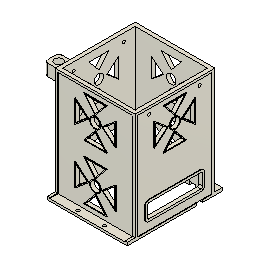
STRUCTURE-V1.0.1 (Autodesk Fusion 360 design; units mm, degrees)
Autodesk Fusion 360 part; units mm, degrees
note: some values were not read from the file. Set by a fixed rule: which sketch regions a step uses.
(part 1 of 2)
sketch "Sketch1" plane through (0, 0, 0) normal (0, 1, 0) x (1, 0, 0)
  line L0 (0, 0) -> (45, 0)
  line L1 (45, 0) -> (45, -45)
  line L2 (45, -45) -> (0, -45)
  line L3 (0, -45) -> (0, 0)
  line L4 (47.5, 2.5) -> (47.5, -47.5)
  line L5 (47.5, -47.5) -> (-2.5, -47.5)
  line L6 (-2.5, -47.5) -> (-2.5, 2.5)
  line L7 (-2.5, 2.5) -> (47.5, 2.5)
  dimension "d1" = 45
  dimension "d2" = 45
  dimension "d3" = -2.5
  constraint horizontal L0
  constraint vertical L1
  constraint horizontal L2
  constraint vertical L3
  constraint coincident L0.start L3.end
  measures "d1" distance of L0.start L0.end
  measures "d2" distance of L0.start L2.end
extrude "Extrude1" add sketch "Sketch1" along normal blind 70
sketch "Sketch2" plane through (0, 0, 47.5) normal (0, 0, 1) x (1, 0, 0)
  line L0 (-2.5, 0) -> (47.5, 0)
  line L1 (47.5, 0) -> (47.5, 70)
  line L2 (47.5, 70) -> (-2.5, 70)
  line L3 (-2.5, 70) -> (-2.5, 0)
  line L4 (-2.5, 35) -> (47.5, 35) construction
  circle A0 centre (22.5, 52.5) radius 3
  circle A1 centre (22.5, 17.5) radius 3
  line L5 (10, 65) -> (35, 65) construction
  line L6 (35, 65) -> (35, 40) construction
  line L7 (35, 40) -> (10, 40) construction
  line L8 (10, 40) -> (10, 65) construction
  line L9 (35, 52.5) -> (10, 52.5) construction
  line L10 (22.5, 65) -> (22.5, 40) construction
  line L11 (17.5, 57.5) -> (27.5, 57.5) construction
  line L12 (27.5, 57.5) -> (27.5, 47.5) construction
  line L13 (27.5, 47.5) -> (17.5, 47.5) construction
  line L14 (17.5, 47.5) -> (17.5, 57.5) construction
  line L15 (17.5, 22.5) -> (27.5, 22.5) construction
  line L16 (27.5, 22.5) -> (27.5, 12.5) construction
  line L17 (27.5, 12.5) -> (17.5, 12.5) construction
  line L18 (17.5, 12.5) -> (17.5, 22.5) construction
  line L19 (10, 30) -> (35, 30) construction
  line L20 (35, 30) -> (35, 5) construction
  line L21 (35, 5) -> (10, 5) construction
  line L22 (10, 5) -> (10, 30) construction
  line L23 (22.5, 57.5) -> (28.75, 65)
  line L24 (22.5, 57.5) -> (16.25, 65)
  line L25 (27.5, 52.5) -> (35, 58.75)
  line L26 (27.5, 52.5) -> (35, 46.25)
  line L27 (22.5, 47.5) -> (16.25, 40)
  line L28 (22.5, 47.5) -> (28.75, 40)
  line L29 (17.5, 52.5) -> (10, 58.75)
  line L30 (17.5, 52.5) -> (10, 46.25)
  line L31 (22.5, 22.5) -> (16.25, 30)
  line L32 (22.5, 22.5) -> (28.75, 30)
  line L33 (27.5, 17.5) -> (35, 23.75)
  line L34 (27.5, 17.5) -> (35, 11.25)
  line L35 (22.5, 12.5) -> (16.25, 5)
  line L36 (22.5, 12.5) -> (28.75, 5)
  line L37 (17.5, 17.5) -> (10, 23.75)
  line L38 (17.5, 17.5) -> (10, 11.25)
  line L39 (16.25, 65) -> (28.75, 65)
  line L40 (16.25, 5) -> (28.75, 5)
  line L41 (35, 11.25) -> (35, 23.75)
  line L42 (10, 23.75) -> (10, 11.25)
  line L43 (16.25, 30) -> (28.75, 30)
  line L44 (10, 46.25) -> (10, 58.75)
  line L45 (16.25, 40) -> (28.75, 40)
  line L46 (35, 46.25) -> (35, 58.75)
  line L47 (16.25, 65) -> (28.75, 65)
  dimension "d6" = 35
  dimension "d7" = 6
  dimension "d8" = 25
  dimension "d9" = 17.5
  dimension "d10" = 6
  dimension "d11" = 25
  dimension "d12" = 17.5
  dimension "d13" = 25
  dimension "d14" = 25
  dimension "d15" = 12.5
  dimension "d16" = 12.5
  dimension "d17" = 10
  dimension "d18" = 10
  dimension "d19" = 5
  dimension "d20" = 10
  dimension "d21" = 10
  dimension "d22" = 5
  dimension "d23" = 5
  dimension "d24" = 25
  dimension "d25" = 25
  dimension "d26" = 12.5
  dimension "d27" = 12.5
  dimension "d28" = 6.25
  dimension "d30" = 6.25
  dimension "d31" = 6.25
  dimension "d32" = 6.25
  dimension "d33" = 6.25
  dimension "d34" = 6.25
  dimension "d35" = 6.25
  dimension "d36" = 6.25
  dimension "d37" = 6.25
  dimension "d38" = 6.25
  dimension "d39" = 6.25
  dimension "d40" = 6.25
  dimension "d41" = 6.25
  dimension "d42" = 6.25
  dimension "d43" = 6.25
  dimension "d44" = 6.25
  constraint coincident L3 L4.start
  constraint coincident L1 L4.end
  constraint perpendicular L1 L4
  constraint horizontal L5
  constraint vertical L6
  constraint horizontal L7
  constraint vertical L8
  constraint midpoint L6 L9.start
  constraint midpoint L8 L9.end
  constraint midpoint L5 L10.start
  constraint midpoint L7 L10.end
  constraint horizontal L11
  constraint vertical L12
  constraint horizontal L13
  constraint vertical L14
  constraint horizontal L15
  constraint vertical L16
  constraint horizontal L17
  constraint vertical L18
  constraint horizontal L19
  constraint vertical L20
  constraint horizontal L21
  constraint vertical L22
  constraint midpoint L11 L23.start
  constraint coincident L5 L23.end
  constraint coincident L5 L24.end
  constraint midpoint L12 L25.start
  constraint coincident L6 L25.end
  constraint coincident L6 L26.end
  constraint midpoint L13 L27.start
  constraint coincident L7 L27.end
  constraint coincident L7 L28.end
  constraint midpoint L14 L29.start
  constraint coincident L8 L29.end
  constraint coincident L8 L30.end
  constraint midpoint L15 L31.start
  constraint coincident L19 L31.end
  constraint coincident L19 L32.end
  constraint midpoint L16 L33.start
  constraint coincident L20 L33.end
  constraint coincident L20 L34.end
  constraint midpoint L17 L35.start
  constraint coincident L21 L35.end
  constraint coincident L21 L36.end
  constraint midpoint L18 L37.start
  constraint coincident L22 L37.end
  constraint coincident L22 L38.end
  measures "d6" distance of L2 L4
  measures "d7" diameter of A0
  measures "d8" distance of L3 A0.centre
  measures "d9" distance of L2 A0.centre
  measures "d10" diameter of A1
  measures "d11" distance of L3 A1.centre
  measures "d12" distance of L0 A1.centre
  measures "d13" distance of L5.start L5.end
  measures "d14" distance of L5.start L7.end
  measures "d15" distance of A0.centre L8
  measures "d16" distance of A0.centre L5
  measures "d17" distance of L11.start L11.end
  measures "d18" distance of L11.start L13.end
  measures "d19" distance of A0.centre L14
  measures "d20" distance of L15.start L15.end
  measures "d21" distance of L15.start L17.end
  measures "d22" distance of A1.centre L18
  measures "d23" distance of A1.centre L15
  measures "d24" distance of L19.start L19.end
  measures "d25" distance of L19.start L21.end
  measures "d26" distance of A1.centre L19
  measures "d27" distance of A1.centre L22
  measures "d28" distance of L5.end L23.end
  measures "d30" distance of L5.start L24.end
  measures "d31" distance of L5.end L25.end
  measures "d32" distance of L6.end L26.end
  measures "d33" distance of L6.end L28.end
  measures "d34" distance of L7.end L27.end
  measures "d35" distance of L5 L29.end
  measures "d36" distance of L7.end L30.end
  measures "d37" distance of L22 L31.end
  measures "d38" distance of L19.end L32.end
  measures "d39" distance of L19.end L33.end
  measures "d40" distance of L20.end L34.end
  measures "d41" distance of L21.end L35.end
  measures "d42" distance of L20.end L36.end
  measures "d43" distance of L19.start L37.end
  measures "d44" distance of L21.end L38.end
extrude "Extrude2" cut sketch "Sketch2" against normal blind 200 contours A0 | A1 | L23 L24 L39 L47 | L25 L26 L46 | L27 L28 L45 | L29 L30 L44 | L31 L32 L43 | L33 L34 L41 | L35 L36 L40 | L37 L38 L42
sketch "Sketch3" plane through (47.5, 0, 0) normal (1, 0, 0) x (0, 0, -1)
  line L0 (-47.5, 0) -> (2.5, 0)
  line L1 (2.5, 0) -> (2.5, 70)
  line L2 (2.5, 70) -> (-47.5, 70)
  line L3 (-47.5, 70) -> (-47.5, 0)
  line L4 (-47.5, 35) -> (2.5, 35) construction
  circle A0 centre (-22.5, 52.5) radius 3
  circle A1 centre (-22.5, 17.5) radius 3
  line L5 (-27.5, 57.5) -> (-17.5, 57.5) construction
  line L6 (-17.5, 57.5) -> (-17.5, 47.5) construction
  line L7 (-17.5, 47.5) -> (-27.5, 47.5) construction
  line L8 (-27.5, 47.5) -> (-27.5, 57.5) construction
  line L9 (-27.5, 22.5) -> (-17.5, 22.5) construction
  line L10 (-17.5, 22.5) -> (-17.5, 12.5) construction
  line L11 (-17.5, 12.5) -> (-27.5, 12.5) construction
  line L12 (-27.5, 12.5) -> (-27.5, 22.5) construction
  line L13 (-35, 65) -> (-10, 65) construction
  line L14 (-10, 65) -> (-10, 40) construction
  line L15 (-10, 40) -> (-35, 40) construction
  line L16 (-35, 40) -> (-35, 65) construction
  line L17 (-35, 30) -> (-10, 30) construction
  line L18 (-10, 30) -> (-10, 5) construction
  line L19 (-10, 5) -> (-35, 5) construction
  line L20 (-35, 5) -> (-35, 30) construction
  line L21 (-22.5, 22.5) -> (-28.75, 30)
  line L22 (-22.5, 22.5) -> (-16.25, 30)
  line L23 (-17.5, 17.5) -> (-10, 23.75)
  line L24 (-17.5, 17.5) -> (-10, 11.25)
  line L25 (-22.5, 12.5) -> (-28.75, 5)
  line L26 (-22.5, 12.5) -> (-16.25, 5)
  line L27 (-22.5, 17.5) -> (-57, 17.5) construction
  line L28 (-27.5, 17.5) -> (-35, 11.25)
  line L29 (-27.5, 17.5) -> (-35, 23.75)
  line L30 (-22.5, 57.5) -> (-28.75, 65)
  line L31 (-22.5, 57.5) -> (-16.25, 65)
  line L32 (-17.5, 52.5) -> (-10, 58.75)
  line L33 (-17.5, 52.5) -> (-10, 46.25)
  line L34 (-22.5, 47.5) -> (-28.75, 40)
  line L35 (-22.5, 47.5) -> (-16.25, 40)
  line L36 (-27.5, 52.5) -> (-35, 58.75)
  line L37 (-27.5, 52.5) -> (-35, 46.25)
  line L38 (-10, 11.25) -> (-10, 23.75)
  line L39 (-16.25, 5) -> (-28.75, 5)
  line L40 (-35, 11.25) -> (-35, 23.75)
  line L41 (-28.75, 30) -> (-16.25, 30)
  line L42 (-28.75, 65) -> (-16.25, 65)
  line L43 (-10, 58.75) -> (-10, 46.25)
  line L44 (-16.25, 40) -> (-28.75, 40)
  line L45 (-35, 46.25) -> (-35, 58.75)
  dimension "d47" = 6
  dimension "d48" = 6
  dimension "d49" = 17.5
  dimension "d50" = 17.5
  dimension "d51" = 25
  dimension "d52" = 25
  dimension "d53" = 10
  dimension "d54" = 10
  dimension "d55" = 10
  dimension "d56" = 10
  dimension "d57" = 5
  dimension "d58" = 5
  dimension "d59" = 5
  dimension "d60" = 5
  dimension "d61" = 25
  dimension "d62" = 25
  dimension "d63" = 12.5
  dimension "d64" = 12.5
  dimension "d65" = 25
  dimension "d66" = 25
  dimension "d67" = 12.5
  dimension "d68" = 12.5
  dimension "d69" = 6.25
  dimension "d70" = 6.25
  dimension "d71" = 6.25
  dimension "d72" = 6.25
  dimension "d73" = 6.25
  dimension "d74" = 6.25
  dimension "d75" = 6.25
  dimension "d76" = 6.25
  dimension "d77" = 6.25
  dimension "d78" = 6.25
  dimension "d79" = 6.25
  dimension "d80" = 6.25
  dimension "d81" = 6.25
  dimension "d82" = 6.25
  dimension "d83" = 6.25
  dimension "d84" = 6.25
  constraint midpoint L3 L4.start
  constraint midpoint L1 L4.end
  constraint horizontal L5
  constraint vertical L6
  constraint horizontal L7
  constraint vertical L8
  constraint horizontal L9
  constraint vertical L10
  constraint horizontal L11
  constraint vertical L12
  constraint horizontal L13
  constraint vertical L14
  constraint horizontal L15
  constraint vertical L16
  constraint horizontal L17
  constraint vertical L18
  constraint horizontal L19
  constraint vertical L20
  constraint midpoint L9 L21.start
  constraint coincident L17 L21.end
  constraint coincident L17 L22.end
  constraint midpoint L10 L23.start
  constraint coincident L18 L23.end
  constraint coincident L18 L24.end
  constraint midpoint L11 L25.start
  constraint coincident L19 L25.end
  constraint coincident L19 L26.end
  constraint coincident A1.centre L27.start
  constraint perpendicular L12 L27
  constraint midpoint L12 L28.start
  constraint coincident L20 L28.end
  constraint coincident L20 L29.end
  constraint midpoint L5 L30.start
  constraint coincident L13 L30.end
  constraint coincident L13 L31.end
  constraint midpoint L6 L32.start
  constraint coincident L14 L32.end
  constraint coincident L14 L33.end
  constraint midpoint L7 L34.start
  constraint coincident L15 L34.end
  constraint coincident L15 L35.end
  constraint midpoint L8 L36.start
  constraint coincident L16 L36.end
  constraint coincident L16 L37.end
  measures "d47" diameter of A0
  measures "d48" diameter of A1
  measures "d49" distance of L2 A0.centre
  measures "d50" distance of L0 A1.centre
  measures "d51" distance of L1 A0.centre
  measures "d52" distance of L1 A1.centre
  measures "d53" distance of L5.start L5.end
  measures "d54" distance of L5.start L7.end
  measures "d55" distance of L9.start L9.end
  measures "d56" distance of L9.start L11.end
  measures "d57" distance of A0.centre L8
  measures "d58" distance of A0.centre L5
  measures "d59" distance of A1.centre L9
  measures "d60" distance of A1.centre L10
  measures "d61" distance of L13.start L13.end
  measures "d62" distance of L13.start L15.end
  measures "d63" distance of A0.centre L13
  measures "d64" distance of A0.centre L16
  measures "d65" distance of L17.start L17.end
  measures "d66" distance of L17.start L19.end
  measures "d67" distance of A1.centre L20
  measures "d68" distance of A1.centre L17
  measures "d69" distance of L17.start L21.end
  measures "d70" distance of L17.end L22.end
  measures "d71" distance of L17.end L23.end
  measures "d72" distance of L18.end L24.end
  measures "d73" distance of L19.end L25.end
  measures "d74" distance of L18.end L26.end
  measures "d75" distance of L19.end L28.end
  measures "d76" distance of L17.start L29.end
  measures "d77" distance of L13.start L30.end
  measures "d78" distance of L13.end L31.end
  measures "d79" distance of L13.end L32.end
  measures "d80" distance of L14.end L33.end
  measures "d81" distance of L15.end L34.end
  measures "d82" distance of L14.end L35.end
  measures "d83" distance of L13.start L36.end
  measures "d84" distance of L15.end L37.end
extrude "Extrude8" cut sketch "Sketch3" against normal blind 200 contours A0 | L30 L31 L42 | L32 L33 L43 | L34 L35 L44 | L36 L37 L45
extrude "Extrude4" cut 1 faces at (45, 13.3333, 20.4167) along direction (1, 0, 0) blind 0.5
extrude "Extrude5" cut 1 faces at (42, 31.25, 0) along direction (0, 0, -1) blind 0.5
extrude "Extrude6" cut 1 faces at (42, 31.25, 45) along direction (0, 0, 1) blind 0.5
extrude "Extrude7" cut 1 faces at (0, 13.3333, 20.4167) along direction (-1, 0, 0) blind 0.5
sketch "Sketch4" plane through (47.5, 0, 0) normal (1, 0, 0) x (0, 0, -1)
  line L0 (-10, 58.75) -> (-10, 46.25)
  line L1 (-10, 46.25) -> (-17.5, 52.5)
  line L2 (-17.5, 52.5) -> (-10, 58.75)
  line L3 (-35, 46.25) -> (-35, 58.75)
  line L4 (-35, 58.75) -> (-27.5, 52.5)
  line L5 (-27.5, 52.5) -> (-35, 46.25)
  line L6 (-16.25, 40) -> (-28.75, 40)
  line L7 (-28.75, 40) -> (-22.5, 47.5)
  line L8 (-22.5, 47.5) -> (-16.25, 40)
  line L9 (-28.75, 65) -> (-16.25, 65)
  line L10 (-16.25, 65) -> (-22.5, 57.5)
  line L11 (-22.5, 57.5) -> (-28.75, 65)
  circle A0 centre (-22.5, 52.5) radius 3
  line L12 (-47.5, 0) -> (2.5, 0)
  line L13 (2.5, 0) -> (2.5, 70)
  line L14 (2.5, 70) -> (-47.5, 70)
  line L15 (-47.5, 70) -> (-47.5, 0)
  line L16 (-40, 20) -> (-5, 20)
  line L17 (-5, 20) -> (-5, 10)
  line L18 (-5, 10) -> (-40, 10)
  line L19 (-40, 10) -> (-40, 20)
  dimension "d105" = 35
  dimension "d106" = 10
  dimension "d107" = 10
  dimension "d108" = 7.5
  constraint horizontal L16
  constraint vertical L17
  constraint horizontal L18
  constraint vertical L19
  measures "d105" distance of L16.start L16.end
  measures "d106" distance of L16.start L18.end
  measures "d107" distance of L12 L18
  measures "d108" distance of L15 L19
extrude "Extrude9" cut sketch "Sketch4" against normal blind 200 contours L16 L17 L18 L19
sketch "Sketch5" plane through (47.5, 0, 0) normal (1, 0, 0) x (0, 0, -1)
  line L0 (-5, 20) -> (-5, 10)
  line L1 (-5, 10) -> (-40, 10)
  line L2 (-40, 10) -> (-40, 20)
  line L3 (-40, 20) -> (-5, 20)
  line L4 (-10, 58.75) -> (-10, 46.25)
  line L5 (-10, 46.25) -> (-17.5, 52.5)
  line L6 (-17.5, 52.5) -> (-10, 58.75)
  line L7 (-35, 46.25) -> (-35, 58.75)
  line L8 (-35, 58.75) -> (-27.5, 52.5)
  line L9 (-27.5, 52.5) -> (-35, 46.25)
  line L10 (-16.25, 40) -> (-28.75, 40)
  line L11 (-28.75, 40) -> (-22.5, 47.5)
  line L12 (-22.5, 47.5) -> (-16.25, 40)
  line L13 (-28.75, 65) -> (-16.25, 65)
  line L14 (-16.25, 65) -> (-22.5, 57.5)
  line L15 (-22.5, 57.5) -> (-28.75, 65)
  circle A0 centre (-22.5, 52.5) radius 3
  line L16 (-47.5, 0) -> (2.5, 0)
  line L17 (2.5, 0) -> (2.5, 70)
  line L18 (2.5, 70) -> (-47.5, 70)
  line L19 (-47.5, 70) -> (-47.5, 0)
  circle A1 centre (-38.5, 65) radius 0.9
  circle A2 centre (-6.5, 65) radius 0.9
  dimension "d111" = 1.8
  dimension "d112" = 1.8
  dimension "d113" = 5
  dimension "d114" = 5
  dimension "d115" = 9
  dimension "d116" = 9
  measures "d111" diameter of A1
  measures "d112" diameter of A2
  measures "d113" distance of L18 A1.centre
  measures "d114" distance of L18 A2.centre
  measures "d115" distance of L19 A1.centre
  measures "d116" distance of L17 A2.centre
extrude "Extrude10" cut sketch "Sketch5" against normal blind 200 contours A1 | A2
extrude "Extrude11" add 1 faces at (46.8333, 20, 28.3333) along direction (0, -1, 0) blind 3
extrude "Extrude12" cut 1 faces at (46.8333, 10, 16.6667) along direction (0, -1, 0) blind 2
sketch "Sketch6" plane through (-2.5, 0, 0) normal (-1, 0, 0) x (0, 0, 1)
  circle A0 centre (38.5, 65) radius 0.9
  circle A1 centre (6.5, 65) radius 0.9
  line L0 (5, 10) -> (5, 20)
  line L1 (5, 20) -> (40, 20)
  line L2 (40, 20) -> (40, 10)
  line L3 (40, 10) -> (5, 10)
  line L4 (10, 46.25) -> (10, 58.75)
  line L5 (10, 58.75) -> (17.5, 52.5)
  line L6 (17.5, 52.5) -> (10, 46.25)
  line L7 (35, 58.75) -> (35, 46.25)
  line L8 (35, 46.25) -> (27.5, 52.5)
  line L9 (27.5, 52.5) -> (35, 58.75)
  line L10 (28.75, 40) -> (16.25, 40)
  line L11 (16.25, 40) -> (22.5, 47.5)
  line L12 (22.5, 47.5) -> (28.75, 40)
  line L13 (16.25, 65) -> (28.75, 65)
  line L14 (28.75, 65) -> (22.5, 57.5)
  line L15 (22.5, 57.5) -> (16.25, 65)
  circle A2 centre (22.5, 52.5) radius 3
  line L16 (-2.5, 0) -> (47.5, 0)
  line L17 (47.5, 0) -> (47.5, 70)
  line L18 (47.5, 70) -> (-2.5, 70)
  line L19 (-2.5, 70) -> (-2.5, 0)
  line L20 (40, 20) -> (28, 20)
  line L21 (28, 20) -> (28, 25)
  line L22 (28, 25) -> (40, 25)
  line L23 (40, 25) -> (40, 20)
  dimension "d123" = 12
  dimension "d124" = 5
  constraint horizontal L20
  constraint vertical L21
  constraint horizontal L22
  constraint vertical L23
  constraint coincident L1.end L2.start
  measures "d123" distance of L1.end L20.end
  measures "d124" distance of L1.end L22.end
extrude "Extrude13" cut sketch "Sketch6" against normal blind 5 contours L1 L20 L21 L22 L23
fillet "Fillet8" radius 1 1 edges at (-1.5, 10, 5)
fillet "Fillet9" radius 1 3 edges at (-1.5, 20, 5) (-1.5, 20, 28) (-1.5, 25, 28)
fillet "Fillet10" radius 1 2 edges at (-1.5, 25, 40) (-1.5, 10, 40)
fillet "Fillet11" radius 1 1 edges at (46.5, 17, 40)
fillet "Fillet12" radius 1 1 edges at (46.5, 8, 40)
fillet "Fillet13" radius 1 1 edges at (46.5, 17, 5)
fillet "Fillet14" radius 1 1 edges at (46.5, 8, 5)
sketch "Sketch8" plane through (47.5, 0, 0) normal (1, 0, 0) x (0, 0, -1)
  line L0 (-47.5, 0) -> (2.5, 0)
  line L1 (2.5, 0) -> (2.5, 70)
  line L2 (2.5, 70) -> (-47.5, 70)
  line L3 (-47.5, 70) -> (-47.5, 0)
  circle A0 centre (-22.5, 52.5) radius 3
  line L4 (-28.75, 65) -> (-16.25, 65)
  line L5 (-16.25, 65) -> (-22.5, 57.5)
  line L6 (-22.5, 57.5) -> (-28.75, 65)
  line L7 (-16.25, 40) -> (-28.75, 40)
  line L8 (-28.75, 40) -> (-22.5, 47.5)
  line L9 (-22.5, 47.5) -> (-16.25, 40)
  line L10 (-35, 46.25) -> (-35, 58.75)
  line L11 (-35, 58.75) -> (-27.5, 52.5)
  line L12 (-27.5, 52.5) -> (-35, 46.25)
  line L13 (-10, 58.75) -> (-10, 46.25)
  line L14 (-10, 46.25) -> (-17.5, 52.5)
  line L15 (-17.5, 52.5) -> (-10, 58.75)
  line L16 (-5, 16) -> (-5, 9)
  arc A1 (-6, 8) -> (-5, 9) centre (-6, 9) ccw
  line L17 (-6, 8) -> (-39, 8)
  arc A2 (-40, 9) -> (-39, 8) centre (-39, 9) ccw
  line L18 (-40, 9) -> (-40, 16)
  arc A3 (-39, 17) -> (-40, 16) centre (-39, 16) ccw
  line L19 (-39, 17) -> (-6, 17)
  arc A4 (-5, 16) -> (-6, 17) centre (-6, 16) ccw
  circle A5 centre (-6.5, 65) radius 0.9
  circle A6 centre (-38.5, 65) radius 0.9
  line L20 (1, 1.5) -> (1, 68.5)
  line L21 (1, 68.5) -> (-46, 68.5)
  line L22 (-46, 68.5) -> (-46, 1.5)
  line L23 (-46, 1.5) -> (1, 1.5)
  dimension "d152" = -1.5
extrude "Extrude15" add sketch "Sketch8" along normal blind 0.35 contours L0 L1 L2 L3
sketch "Sketch10" plane through (0, 0, -2.5) normal (0, 0, -1) x (-1, 0, 0)
  circle A0 centre (-22.5, 17.5) radius 3
  line L0 (-35, 46.25) -> (-35, 58.75)
  line L1 (-35, 58.75) -> (-27.5, 52.5)
  line L2 (-27.5, 52.5) -> (-35, 46.25)
  circle A1 centre (-22.5, 52.5) radius 3
  line L3 (-16.25, 40) -> (-28.75, 40)
  line L4 (-28.75, 40) -> (-22.5, 47.5)
  line L5 (-22.5, 47.5) -> (-16.25, 40)
  line L6 (-16.25, 5) -> (-28.75, 5)
  line L7 (-28.75, 5) -> (-22.5, 12.5)
  line L8 (-22.5, 12.5) -> (-16.25, 5)
  line L9 (-10, 23.75) -> (-10, 11.25)
  line L10 (-10, 11.25) -> (-17.5, 17.5)
  line L11 (-17.5, 17.5) -> (-10, 23.75)
  line L12 (-10, 58.75) -> (-10, 46.25)
  line L13 (-10, 46.25) -> (-17.5, 52.5)
  line L14 (-17.5, 52.5) -> (-10, 58.75)
  line L15 (-28.75, 65) -> (-16.25, 65)
  line L16 (-16.25, 65) -> (-22.5, 57.5)
  line L17 (-22.5, 57.5) -> (-28.75, 65)
  line L18 (-28.75, 30) -> (-16.25, 30)
  line L19 (-16.25, 30) -> (-22.5, 22.5)
  line L20 (-22.5, 22.5) -> (-28.75, 30)
  line L21 (-35, 11.25) -> (-35, 23.75)
  line L22 (-35, 23.75) -> (-27.5, 17.5)
  line L23 (-27.5, 17.5) -> (-35, 11.25)
  line L24 (-47.85, 0) -> (2.5, 0)
  line L25 (2.5, 0) -> (2.5, 70)
  line L26 (2.5, 70) -> (-47.85, 70)
  line L27 (-47.85, 70) -> (-47.85, 0)
  line L28 (1, 1.5) -> (1, 68.5)
  line L29 (1, 68.5) -> (-46.35, 68.5)
  line L30 (-46.35, 68.5) -> (-46.35, 1.5)
  line L31 (-46.35, 1.5) -> (1, 1.5)
  dimension "d157" = -1.5
extrude "Extrude16" add sketch "Sketch10" along normal blind 0.4 contours L24 L25 L26 L27
sketch "Sketch11" plane through (-2.5, 0, 0) normal (-1, 0, 0) x (0, 0, 1)
  arc A0 (27, 20) -> (28, 21) centre (27, 21) ccw
  arc A1 (29, 25) -> (28, 24) centre (29, 24) ccw
  line L0 (29, 25) -> (39, 25)
  arc A2 (40, 24) -> (39, 25) centre (39, 24) ccw
  line L1 (40, 24) -> (40, 11)
  arc A3 (39, 10) -> (40, 11) centre (39, 11) ccw
  line L2 (39, 10) -> (6, 10)
  arc A4 (5, 11) -> (6, 10) centre (6, 11) ccw
  line L3 (5, 11) -> (5, 19)
  arc A5 (6, 20) -> (5, 19) centre (6, 19) ccw
  line L4 (6, 20) -> (27, 20)
  line L5 (-2.9, 0) -> (47.5, 0)
  line L6 (47.5, 0) -> (47.5, 70)
  line L7 (47.5, 70) -> (-2.9, 70)
  line L8 (-2.9, 70) -> (-2.9, 0)
  circle A6 centre (22.5, 52.5) radius 3
  line L9 (16.25, 65) -> (28.75, 65)
  line L10 (28.75, 65) -> (22.5, 57.5)
  line L11 (22.5, 57.5) -> (16.25, 65)
  line L12 (28.75, 40) -> (16.25, 40)
  line L13 (16.25, 40) -> (22.5, 47.5)
  line L14 (22.5, 47.5) -> (28.75, 40)
  line L15 (35, 58.75) -> (35, 46.25)
  line L16 (35, 46.25) -> (27.5, 52.5)
  line L17 (27.5, 52.5) -> (35, 58.75)
  line L18 (10, 46.25) -> (10, 58.75)
  line L19 (10, 58.75) -> (17.5, 52.5)
  line L20 (17.5, 52.5) -> (10, 46.25)
  circle A7 centre (6.5, 65) radius 0.9
  circle A8 centre (38.5, 65) radius 0.9
  line L21 (46, 1.5) -> (46, 68.5)
  line L22 (46, 68.5) -> (-1.4, 68.5)
  line L23 (-1.4, 68.5) -> (-1.4, 1.5)
  line L24 (-1.4, 1.5) -> (46, 1.5)
  line L25 (28, 21) -> (28, 24)
  dimension "d160" = -1.5
extrude "Extrude17" add sketch "Sketch11" along normal blind 0.35 contours L5 L6 L7 L8
sketch "Sketch12" plane through (0, 0, 47.5) normal (0, 0, 1) x (1, 0, 0)
  circle A0 centre (22.5, 17.5) radius 3
  line L0 (35, 58.75) -> (35, 46.25)
  line L1 (35, 46.25) -> (27.5, 52.5)
  line L2 (27.5, 52.5) -> (35, 58.75)
  circle A1 centre (22.5, 52.5) radius 3
  line L3 (28.75, 40) -> (16.25, 40)
  line L4 (16.25, 40) -> (22.5, 47.5)
  line L5 (22.5, 47.5) -> (28.75, 40)
  line L6 (28.75, 5) -> (16.25, 5)
  line L7 (16.25, 5) -> (22.5, 12.5)
  line L8 (22.5, 12.5) -> (28.75, 5)
  line L9 (10, 11.25) -> (10, 23.75)
  line L10 (10, 23.75) -> (17.5, 17.5)
  line L11 (17.5, 17.5) -> (10, 11.25)
  line L12 (10, 46.25) -> (10, 58.75)
  line L13 (10, 58.75) -> (17.5, 52.5)
  line L14 (17.5, 52.5) -> (10, 46.25)
  line L15 (16.25, 65) -> (28.75, 65)
  line L16 (28.75, 65) -> (22.5, 57.5)
  line L17 (22.5, 57.5) -> (16.25, 65)
  line L18 (16.25, 30) -> (28.75, 30)
  line L19 (28.75, 30) -> (22.5, 22.5)
  line L20 (22.5, 22.5) -> (16.25, 30)
  line L21 (35, 23.75) -> (35, 11.25)
  line L22 (35, 11.25) -> (27.5, 17.5)
  line L23 (27.5, 17.5) -> (35, 23.75)
  line L24 (-2.85, 0) -> (47.85, 0)
  line L25 (47.85, 0) -> (47.85, 70)
  line L26 (47.85, 70) -> (-2.85, 70)
  line L27 (-2.85, 70) -> (-2.85, 0)
  line L28 (46.35, 1.5) -> (46.35, 68.5)
  line L29 (46.35, 68.5) -> (-1.35, 68.5)
  line L30 (-1.35, 68.5) -> (-1.35, 1.5)
  line L31 (-1.35, 1.5) -> (46.35, 1.5)
  dimension "d163" = -1.5
extrude "Extrude18" add sketch "Sketch12" along normal blind 0.35 contours L24 L25 L26 L27
sketch "Sketch17" plane through (0, 0, -2.9) normal (0, 0, -1) x (-1, 0, 0)
  line L0 (1, 1.5) -> (-46.35, 1.5)
  line L1 (-46.35, 1.5) -> (-46.35, 68.5)
  line L2 (-46.35, 68.5) -> (1, 68.5)
  line L3 (1, 68.5) -> (1, 1.5)
  line L4 (-47.85, 70) -> (-47.85, 0)
  line L5 (-47.85, 0) -> (2.85, 0)
  line L6 (2.85, 0) -> (2.85, 70)
  line L7 (2.85, 70) -> (-47.85, 70)
  line L8 (-37.85, 0) -> (-33.85, 0)
  line L9 (-33.85, 0) -> (-33.85, 1.5)
  line L10 (-33.85, 1.5) -> (-37.85, 1.5)
  line L11 (-37.85, 1.5) -> (-37.85, 0)
  dimension "d198" = 4
  dimension "d199" = 1.5
  dimension "d200" = 10
  constraint horizontal L8
  constraint vertical L9
  constraint horizontal L10
  constraint vertical L11
  constraint coincident L5 L8.start
  measures "d198" distance of L8.start L8.end
  measures "d199" distance of L8.start L10.end
  measures "d200" distance of L4 L11
extrude "Extrude23" cut sketch "Sketch17" against normal blind 5 contours L0 L5 L8 L9 L10 L11
extrude "Extrude24" cut 1 faces at (35.1833, 1.5, -1.1667) along direction (0, 1, 0) blind 0.5
sketch "Sketch18" plane through (47.85, 0, 0) normal (1, 0, 0) x (0, 0, -1)
  line L0 (1, 1.5) -> (-46, 1.5)
  line L1 (-46, 1.5) -> (-46, 68.5)
  line L2 (-46, 68.5) -> (1, 68.5)
  line L3 (1, 68.5) -> (1, 1.5)
  line L4 (-47.85, 0) -> (2.9, 0)
  line L5 (2.9, 0) -> (2.9, 70)
  line L6 (2.9, 70) -> (-47.85, 70)
  line L7 (-47.85, 70) -> (-47.85, 0)
  line L8 (-5, 0) -> (-9, 0)
  line L9 (-9, 0) -> (-9, 1.5)
  line L10 (-9, 1.5) -> (-5, 1.5)
  line L11 (-5, 1.5) -> (-5, 0)
  dimension "d205" = 4
  dimension "d206" = 1.5
  constraint horizontal L8
  constraint vertical L9
  constraint horizontal L10
  constraint vertical L11
  constraint coincident L4 L8.start
  measures "d205" distance of L8.start L8.end
  measures "d206" distance of L8 L10
extrude "Extrude25" cut sketch "Sketch18" against normal blind 5 contours L0 L4 L8 L9 L10 L11
sketch "Sketch19" plane through (47.5, 0, 0) normal (1, 0, 0) x (0, 0, -1)
  line L0 (1, 1.5) -> (1, 68.5)
  line L1 (1, 68.5) -> (-46, 68.5)
  line L2 (-46, 68.5) -> (-46, 1.5)
  line L3 (-46, 1.5) -> (-9, 1.5)
  line L4 (-9, 1.5) -> (-5, 1.5)
  line L5 (-5, 1.5) -> (1, 1.5)
  line L6 (-5, 16) -> (-5, 9)
  arc A0 (-6, 8) -> (-5, 9) centre (-6, 9) ccw
  line L7 (-6, 8) -> (-39, 8)
  arc A1 (-40, 9) -> (-39, 8) centre (-39, 9) ccw
  line L8 (-40, 9) -> (-40, 16)
  arc A2 (-39, 17) -> (-40, 16) centre (-39, 16) ccw
  line L9 (-39, 17) -> (-6, 17)
  arc A3 (-5, 16) -> (-6, 17) centre (-6, 16) ccw
  circle A4 centre (-6.5, 65) radius 0.9
  circle A5 centre (-38.5, 65) radius 0.9
  arc A6 (-41.5, 9) -> (-39, 6.5) centre (-39, 9) ccw
  line L10 (-6, 6.5) -> (-39, 6.5)
  arc A7 (-6, 6.5) -> (-3.5, 9) centre (-6, 9) ccw
  line L11 (-3.5, 16) -> (-3.5, 9)
  arc A8 (-3.5, 16) -> (-6, 18.5) centre (-6, 16) ccw
  line L12 (-39, 18.5) -> (-6, 18.5)
  arc A9 (-39, 18.5) -> (-41.5, 16) centre (-39, 16) ccw
  line L13 (-41.5, 9) -> (-41.5, 16)
  circle A10 centre (-22.5, 52.5) radius 3
  line L14 (-28.75, 65) -> (-16.25, 65)
  line L15 (-16.25, 65) -> (-22.5, 57.5)
  line L16 (-22.5, 57.5) -> (-28.75, 65)
  line L17 (-16.25, 40) -> (-28.75, 40)
  line L18 (-28.75, 40) -> (-22.5, 47.5)
  line L19 (-22.5, 47.5) -> (-16.25, 40)
  line L20 (-35, 46.25) -> (-35, 58.75)
  line L21 (-35, 58.75) -> (-27.5, 52.5)
  line L22 (-27.5, 52.5) -> (-35, 46.25)
  line L23 (-10, 58.75) -> (-10, 46.25)
  line L24 (-10, 46.25) -> (-17.5, 52.5)
  line L25 (-17.5, 52.5) -> (-10, 58.75)
  dimension "d209" = -1.5
extrude "Extrude26" add sketch "Sketch19" along normal blind 0.35 contours A6 L10 A7 L11 A8 L12 A9 L13
sketch "Sketch21" plane through (-2.5, 0, 0) normal (-1, 0, 0) x (0, 0, 1)
  line L0 (46, 1.5) -> (46, 68.5)
  line L1 (46, 68.5) -> (-1.4, 68.5)
  line L2 (-1.4, 68.5) -> (-1.4, 1.5)
  line L3 (-1.4, 1.5) -> (46, 1.5)
  arc A0 (27, 20) -> (28, 21) centre (27, 21) ccw
  line L4 (28, 21) -> (28, 24)
  arc A1 (29, 25) -> (28, 24) centre (29, 24) ccw
  line L5 (29, 25) -> (39, 25)
  arc A2 (40, 24) -> (39, 25) centre (39, 24) ccw
  line L6 (40, 24) -> (40, 11)
  arc A3 (39, 10) -> (40, 11) centre (39, 11) ccw
  line L7 (39, 10) -> (6, 10)
  arc A4 (5, 11) -> (6, 10) centre (6, 11) ccw
  line L8 (5, 11) -> (5, 19)
  arc A5 (6, 20) -> (5, 19) centre (6, 19) ccw
  line L9 (6, 20) -> (27, 20)
  circle A6 centre (6.5, 65) radius 0.9
  circle A7 centre (38.5, 65) radius 0.9
  line L10 (26.5, 21.5) -> (26.5, 24)
  arc A8 (29, 26.5) -> (26.5, 24) centre (29, 24) ccw
  line L11 (29, 26.5) -> (39, 26.5)
  arc A9 (41.5, 24) -> (39, 26.5) centre (39, 24) ccw
  line L12 (41.5, 24) -> (41.5, 11)
  arc A10 (39, 8.5) -> (41.5, 11) centre (39, 11) ccw
  line L13 (39, 8.5) -> (36.5, 8.5)
  line L14 (36.5, 8.5) -> (36.5, 4)
  arc A11 (34, 1.5) -> (36.5, 4) centre (34, 4) ccw
  line L15 (34, 1.5) -> (26, 1.5)
  arc A12 (23.5, 4) -> (26, 1.5) centre (26, 4) ccw
  line L16 (23.5, 4) -> (23.5, 8.5)
  line L17 (23.5, 8.5) -> (6, 8.5)
  arc A13 (3.5, 11) -> (6, 8.5) centre (6, 11) ccw
  line L18 (3.5, 11) -> (3.5, 19)
  arc A14 (6, 21.5) -> (3.5, 19) centre (6, 19) ccw
  line L19 (6, 21.5) -> (26.5, 21.5)
  circle A15 centre (22.5, 52.5) radius 3
  line L20 (16.25, 65) -> (28.75, 65)
  line L21 (28.75, 65) -> (22.5, 57.5)
  line L22 (22.5, 57.5) -> (16.25, 65)
  line L23 (28.75, 40) -> (16.25, 40)
  line L24 (16.25, 40) -> (22.5, 47.5)
  line L25 (22.5, 47.5) -> (28.75, 40)
  line L26 (35, 58.75) -> (35, 46.25)
  line L27 (35, 46.25) -> (27.5, 52.5)
  line L28 (27.5, 52.5) -> (35, 58.75)
  line L29 (10, 46.25) -> (10, 58.75)
  line L30 (10, 58.75) -> (17.5, 52.5)
  line L31 (17.5, 52.5) -> (10, 46.25)
  constraint parallel L4 L10
  constraint concentric A1 A8
  constraint parallel L5 L11
  constraint concentric A2 A9
  constraint parallel L6 L12
  constraint concentric A3 A10
  constraint parallel L7 L13
  constraint concentric A4 A13
  constraint parallel L8 L18
  constraint concentric A5 A14
  constraint parallel L9 L19
  constraint tangent L10 A8
  constraint tangent A9 L12
  constraint tangent A8 L11
  constraint tangent A13 L18
  constraint tangent L12 A10
  constraint tangent L11 A9
  constraint tangent A10 L13
  constraint tangent L14 A11
  constraint tangent A11 L15
  constraint tangent L15 A12
  constraint tangent A12 L16
  constraint tangent L17 A13
  constraint tangent L18 A14
  constraint tangent A14 L19
extrude "Extrude28" add sketch "Sketch21" along normal blind 0.35 contours L3 L10 A8 L11 A9 L12 A10 L13 L14 A11 L15 A12 L16 L17 A13 L18 A14 L19
sketch "Sketch22" plane through (0, 0, 47.5) normal (0, 0, 1) x (1, 0, 0)
  line L0 (46.35, 1.5) -> (46.35, 68.5)
  line L1 (46.35, 68.5) -> (-1.35, 68.5)
  line L2 (-1.35, 68.5) -> (-1.35, 1.5)
  line L3 (-1.35, 1.5) -> (46.35, 1.5)
  circle A0 centre (22.5, 17.5) radius 3
  line L4 (35, 58.75) -> (35, 46.25)
  line L5 (35, 46.25) -> (27.5, 52.5)
  line L6 (27.5, 52.5) -> (35, 58.75)
  circle A1 centre (22.5, 52.5) radius 3
  line L7 (28.75, 40) -> (16.25, 40)
  line L8 (16.25, 40) -> (22.5, 47.5)
  line L9 (22.5, 47.5) -> (28.75, 40)
  line L10 (28.75, 5) -> (16.25, 5)
  line L11 (16.25, 5) -> (22.5, 12.5)
  line L12 (22.5, 12.5) -> (28.75, 5)
  line L13 (10, 11.25) -> (10, 23.75)
  line L14 (10, 23.75) -> (17.5, 17.5)
  line L15 (17.5, 17.5) -> (10, 11.25)
  line L16 (10, 46.25) -> (10, 58.75)
  line L17 (10, 58.75) -> (17.5, 52.5)
  line L18 (17.5, 52.5) -> (10, 46.25)
  line L19 (16.25, 65) -> (28.75, 65)
  line L20 (28.75, 65) -> (22.5, 57.5)
  line L21 (22.5, 57.5) -> (16.25, 65)
  line L22 (16.25, 30) -> (28.75, 30)
  line L23 (28.75, 30) -> (22.5, 22.5)
  line L24 (22.5, 22.5) -> (16.25, 30)
  line L25 (35, 23.75) -> (35, 11.25)
  line L26 (35, 11.25) -> (27.5, 17.5)
  line L27 (27.5, 17.5) -> (35, 23.75)
  line L28 (9.5, 59.8175) -> (18.281, 52.5)
  line L29 (18.281, 52.5) -> (9.5, 45.1825)
  line L30 (9.5, 45.1825) -> (9.5, 59.8175)
  line L31 (29.8175, 65.5) -> (22.5, 56.719)
  line L32 (22.5, 56.719) -> (15.1825, 65.5)
  line L33 (15.1825, 65.5) -> (29.8175, 65.5)
  line L34 (35.5, 45.1825) -> (26.719, 52.5)
  line L35 (26.719, 52.5) -> (35.5, 59.8175)
  line L36 (35.5, 59.8175) -> (35.5, 45.1825)
  line L37 (22.5, 48.281) -> (29.8175, 39.5)
  line L38 (29.8175, 39.5) -> (15.1825, 39.5)
  line L39 (15.1825, 39.5) -> (22.5, 48.281)
  line L40 (29.8175, 30.5) -> (22.5, 21.719)
  line L41 (22.5, 21.719) -> (15.1825, 30.5)
  line L42 (15.1825, 30.5) -> (29.8175, 30.5)
  line L43 (35.5, 10.1825) -> (26.719, 17.5)
  line L44 (26.719, 17.5) -> (35.5, 24.8175)
  line L45 (35.5, 24.8175) -> (35.5, 10.1825)
  line L46 (9.5, 24.8175) -> (18.281, 17.5)
  line L47 (18.281, 17.5) -> (9.5, 10.1825)
  line L48 (9.5, 10.1825) -> (9.5, 24.8175)
  line L49 (29.8175, 4.5) -> (15.1825, 4.5)
  line L50 (15.1825, 4.5) -> (22.5, 13.281)
  line L51 (22.5, 13.281) -> (29.8175, 4.5)
  dimension "d218" = -0.5
  dimension "d219" = -0.5
  dimension "d220" = -0.5
  dimension "d221" = -0.5
  dimension "d222" = -0.5
  dimension "d223" = -0.5
  dimension "d224" = -0.5
  dimension "d225" = -0.5
extrude "Extrude29" add sketch "Sketch22" along normal blind 0.35 contours L28 L29 L30 | L31 L32 L33 | L34 L35 L36 | L37 L38 L39 | L40 L41 L42 | L43 L44 L45 | L46 L47 L48 | L49 L50 L51
sketch "Sketch23" plane through (-2.5, 0, 0) normal (-1, 0, 0) x (0, 0, 1)
  circle A0 centre (38.5, 65) radius 0.9
  circle A1 centre (6.5, 65) radius 0.9
  line L0 (10, 46.25) -> (10, 58.75)
  line L1 (10, 58.75) -> (17.5, 52.5)
  line L2 (17.5, 52.5) -> (10, 46.25)
  line L3 (35, 58.75) -> (35, 46.25)
  line L4 (35, 46.25) -> (27.5, 52.5)
  line L5 (27.5, 52.5) -> (35, 58.75)
  line L6 (28.75, 40) -> (16.25, 40)
  line L7 (16.25, 40) -> (22.5, 47.5)
  line L8 (22.5, 47.5) -> (28.75, 40)
  line L9 (16.25, 65) -> (28.75, 65)
  line L10 (28.75, 65) -> (22.5, 57.5)
  line L11 (22.5, 57.5) -> (16.25, 65)
  circle A2 centre (22.5, 52.5) radius 3
  arc A3 (23.5, 4) -> (26, 1.5) centre (26, 4) ccw
  line L12 (23.5, 4) -> (23.5, 8.5)
  line L13 (23.5, 8.5) -> (6, 8.5)
  arc A4 (3.5, 11) -> (6, 8.5) centre (6, 11) ccw
  line L14 (3.5, 11) -> (3.5, 19)
  arc A5 (6, 21.5) -> (3.5, 19) centre (6, 19) ccw
  line L15 (6, 21.5) -> (26.5, 21.5)
  line L16 (26.5, 21.5) -> (26.5, 24)
  arc A6 (29, 26.5) -> (26.5, 24) centre (29, 24) ccw
  line L17 (29, 26.5) -> (39, 26.5)
  arc A7 (41.5, 24) -> (39, 26.5) centre (39, 24) ccw
  line L18 (41.5, 24) -> (41.5, 11)
  arc A8 (39, 8.5) -> (41.5, 11) centre (39, 11) ccw
  line L19 (39, 8.5) -> (36.5, 8.5)
  line L20 (36.5, 8.5) -> (36.5, 4)
  arc A9 (34, 1.5) -> (36.5, 4) centre (34, 4) ccw
  line L21 (34, 1.5) -> (46, 1.5)
  line L22 (46, 1.5) -> (46, 68.5)
  line L23 (46, 68.5) -> (-1.4, 68.5)
  line L24 (-1.4, 68.5) -> (-1.4, 1.5)
  line L25 (-1.4, 1.5) -> (26, 1.5)
  line L26 (15.1825, 65.5) -> (29.8175, 65.5)
  line L27 (29.8175, 65.5) -> (22.5, 56.719)
  line L28 (22.5, 56.719) -> (15.1825, 65.5)
  line L29 (35.5, 45.1825) -> (26.719, 52.5)
  line L30 (26.719, 52.5) -> (35.5, 59.8175)
  line L31 (35.5, 59.8175) -> (35.5, 45.1825)
  line L32 (15.1825, 39.5) -> (22.5, 48.281)
  line L33 (22.5, 48.281) -> (29.8175, 39.5)
  line L34 (29.8175, 39.5) -> (15.1825, 39.5)
  line L35 (18.281, 52.5) -> (9.5, 45.1825)
  line L36 (9.5, 45.1825) -> (9.5, 59.8175)
  line L37 (9.5, 59.8175) -> (18.281, 52.5)
  dimension "d228" = -0.5
  dimension "d229" = -0.5
  dimension "d230" = -0.5
  dimension "d231" = -0.5
sketch "Sketch24" plane through (0, 0, -2.5) normal (0, 0, -1) x (-1, 0, 0)
  line L0 (-35, 11.25) -> (-35, 23.75)
  line L1 (-35, 23.75) -> (-27.5, 17.5)
  line L2 (-27.5, 17.5) -> (-35, 11.25)
  line L3 (-28.75, 30) -> (-16.25, 30)
  line L4 (-16.25, 30) -> (-22.5, 22.5)
  line L5 (-22.5, 22.5) -> (-28.75, 30)
  line L6 (-28.75, 65) -> (-16.25, 65)
  line L7 (-16.25, 65) -> (-22.5, 57.5)
  line L8 (-22.5, 57.5) -> (-28.75, 65)
  line L9 (-10, 58.75) -> (-10, 46.25)
  line L10 (-10, 46.25) -> (-17.5, 52.5)
  line L11 (-17.5, 52.5) -> (-10, 58.75)
  line L12 (-10, 23.75) -> (-10, 11.25)
  line L13 (-10, 11.25) -> (-17.5, 17.5)
  line L14 (-17.5, 17.5) -> (-10, 23.75)
  line L15 (-16.25, 5) -> (-28.75, 5)
  line L16 (-28.75, 5) -> (-22.5, 12.5)
  line L17 (-22.5, 12.5) -> (-16.25, 5)
  line L18 (-16.25, 40) -> (-28.75, 40)
  line L19 (-28.75, 40) -> (-22.5, 47.5)
  line L20 (-22.5, 47.5) -> (-16.25, 40)
  circle A0 centre (-22.5, 52.5) radius 3
  line L21 (-35, 46.25) -> (-35, 58.75)
  line L22 (-35, 58.75) -> (-27.5, 52.5)
  line L23 (-27.5, 52.5) -> (-35, 46.25)
  circle A1 centre (-22.5, 17.5) radius 3
  line L24 (-37.85, 1.5) -> (-37.85, 2)
  line L25 (-37.85, 2) -> (-33.85, 2)
  line L26 (-33.85, 2) -> (-33.85, 1.5)
  line L27 (-33.85, 1.5) -> (1, 1.5)
  line L28 (1, 1.5) -> (1, 68.5)
  line L29 (1, 68.5) -> (-46.35, 68.5)
  line L30 (-46.35, 68.5) -> (-46.35, 1.5)
  line L31 (-46.35, 1.5) -> (-37.85, 1.5)
  line L32 (-15.1825, 65.5) -> (-22.5, 56.719)
  line L33 (-22.5, 56.719) -> (-29.8175, 65.5)
  line L34 (-29.8175, 65.5) -> (-15.1825, 65.5)
  line L35 (-26.719, 52.5) -> (-35.5, 45.1825)
  line L36 (-35.5, 45.1825) -> (-35.5, 59.8175)
  line L37 (-35.5, 59.8175) -> (-26.719, 52.5)
  line L38 (-29.8175, 39.5) -> (-22.5, 48.281)
  line L39 (-22.5, 48.281) -> (-15.1825, 39.5)
  line L40 (-15.1825, 39.5) -> (-29.8175, 39.5)
  line L41 (-9.5, 59.8175) -> (-9.5, 45.1825)
  line L42 (-9.5, 45.1825) -> (-18.281, 52.5)
  line L43 (-18.281, 52.5) -> (-9.5, 59.8175)
  line L44 (-29.8175, 30.5) -> (-15.1825, 30.5)
  line L45 (-15.1825, 30.5) -> (-22.5, 21.719)
  line L46 (-22.5, 21.719) -> (-29.8175, 30.5)
  line L47 (-35.5, 24.8175) -> (-26.719, 17.5)
  line L48 (-26.719, 17.5) -> (-35.5, 10.1825)
  line L49 (-35.5, 10.1825) -> (-35.5, 24.8175)
  line L50 (-9.5, 24.8175) -> (-9.5, 10.1825)
  line L51 (-9.5, 10.1825) -> (-18.281, 17.5)
  line L52 (-18.281, 17.5) -> (-9.5, 24.8175)
  line L53 (-29.8175, 4.5) -> (-22.5, 13.281)
  line L54 (-22.5, 13.281) -> (-15.1825, 4.5)
  line L55 (-15.1825, 4.5) -> (-29.8175, 4.5)
  dimension "d234" = -0.5
  dimension "d235" = -0.5
  dimension "d236" = -0.5
  dimension "d237" = -0.5
  dimension "d238" = -0.5
  dimension "d239" = -0.5
  dimension "d240" = -0.5
  dimension "d241" = -0.5
extrude "Extrude31" add sketch "Sketch24" along normal blind 0.35 contours L32 L33 L34 | L35 L36 L37 | L38 L39 L40 | L41 L42 L43 | L44 L45 L46 | L47 L48 L49 | L50 L51 L52 | L53 L54 L55
extrude "Extrude30" add sketch "Sketch23" along normal blind 0.35 contours L26 L27 L28 | L29 L30 L31 | L32 L33 L34 | L35 L36 L37
sketch "Sketch26" plane through (0, 0, 47.5) normal (0, 0, 1) x (1, 0, 0)
  line L0 (35.5, 24.8175) -> (35.5, 10.1825)
  line L1 (35.5, 10.1825) -> (26.719, 17.5)
  line L2 (26.719, 17.5) -> (35.5, 24.8175)
  line L3 (15.1825, 39.5) -> (22.5, 48.281)
  line L4 (22.5, 48.281) -> (29.8175, 39.5)
  line L5 (29.8175, 39.5) -> (15.1825, 39.5)
  line L6 (9.5, 45.1825) -> (9.5, 59.8175)
  line L7 (9.5, 59.8175) -> (18.281, 52.5)
  line L8 (18.281, 52.5) -> (9.5, 45.1825)
  line L9 (15.1825, 30.5) -> (29.8175, 30.5)
  line L10 (29.8175, 30.5) -> (22.5, 21.719)
  line L11 (22.5, 21.719) -> (15.1825, 30.5)
  line L12 (22.5, 13.281) -> (29.8175, 4.5)
  line L13 (29.8175, 4.5) -> (15.1825, 4.5)
  line L14 (15.1825, 4.5) -> (22.5, 13.281)
  line L15 (15.1825, 65.5) -> (29.8175, 65.5)
  line L16 (29.8175, 65.5) -> (22.5, 56.719)
  line L17 (22.5, 56.719) -> (15.1825, 65.5)
  line L18 (35.5, 59.8175) -> (35.5, 45.1825)
  line L19 (35.5, 45.1825) -> (26.719, 52.5)
  line L20 (26.719, 52.5) -> (35.5, 59.8175)
  line L21 (9.5, 10.1825) -> (9.5, 24.8175)
  line L22 (9.5, 24.8175) -> (18.281, 17.5)
  line L23 (18.281, 17.5) -> (9.5, 10.1825)
  line L24 (46.35, 1.5) -> (46.35, 68.5)
  line L25 (46.35, 68.5) -> (-1.35, 68.5)
  line L26 (-1.35, 68.5) -> (-1.35, 1.5)
  line L27 (-1.35, 1.5) -> (46.35, 1.5)
  circle A0 centre (22.5, 17.5) radius 3
  circle A1 centre (22.5, 52.5) radius 3
  circle A2 centre (22.5, 52.5) radius 3.5
  circle A3 centre (22.5, 17.5) radius 3.5
  dimension "d252" = 0.5
  dimension "d253" = 0.5
extrude "Extrude34" add sketch "Sketch26" along normal blind 0.35 contours A2 | A3
sketch "Sketch29" plane through (47.5, 0, 0) normal (1, 0, 0) x (0, 0, -1)
  line L0 (-6, 6.5) -> (-39, 6.5)
  arc A0 (-41.5, 9) -> (-39, 6.5) centre (-39, 9) ccw
  line L1 (-41.5, 9) -> (-41.5, 16)
  arc A1 (-39, 18.5) -> (-41.5, 16) centre (-39, 16) ccw
  line L2 (-39, 18.5) -> (-6, 18.5)
  arc A2 (-3.5, 16) -> (-6, 18.5) centre (-6, 16) ccw
  line L3 (-3.5, 16) -> (-3.5, 9)
  arc A3 (-6, 6.5) -> (-3.5, 9) centre (-6, 9) ccw
  line L4 (1, 1.5) -> (1, 68.5)
  line L5 (1, 68.5) -> (-46, 68.5)
  line L6 (-46, 68.5) -> (-46, 1.5)
  line L7 (-46, 1.5) -> (-9, 1.5)
  line L8 (-9, 1.5) -> (-5, 1.5)
  line L9 (-5, 1.5) -> (1, 1.5)
  circle A4 centre (-22.5, 52.5) radius 3
  line L10 (-28.75, 65) -> (-16.25, 65)
  line L11 (-16.25, 65) -> (-22.5, 57.5)
  line L12 (-22.5, 57.5) -> (-28.75, 65)
  line L13 (-16.25, 40) -> (-28.75, 40)
  line L14 (-28.75, 40) -> (-22.5, 47.5)
  line L15 (-22.5, 47.5) -> (-16.25, 40)
  line L16 (-35, 46.25) -> (-35, 58.75)
  line L17 (-35, 58.75) -> (-27.5, 52.5)
  line L18 (-27.5, 52.5) -> (-35, 46.25)
  line L19 (-10, 58.75) -> (-10, 46.25)
  line L20 (-10, 46.25) -> (-17.5, 52.5)
  line L21 (-17.5, 52.5) -> (-10, 58.75)
  circle A5 centre (-6.5, 65) radius 0.9
  circle A6 centre (-38.5, 65) radius 0.9
  line L22 (-15.1825, 65.5) -> (-22.5, 56.719)
  line L23 (-22.5, 56.719) -> (-29.8175, 65.5)
  line L24 (-29.8175, 65.5) -> (-15.1825, 65.5)
  line L25 (-35.5, 45.1825) -> (-35.5, 59.8175)
  line L26 (-35.5, 59.8175) -> (-26.719, 52.5)
  line L27 (-26.719, 52.5) -> (-35.5, 45.1825)
  line L28 (-9.5, 45.1825) -> (-18.281, 52.5)
  line L29 (-18.281, 52.5) -> (-9.5, 59.8175)
  line L30 (-9.5, 59.8175) -> (-9.5, 45.1825)
  line L31 (-22.5, 48.281) -> (-15.1825, 39.5)
  line L32 (-15.1825, 39.5) -> (-29.8175, 39.5)
  line L33 (-29.8175, 39.5) -> (-22.5, 48.281)
  circle A7 centre (-22.5, 52.5) radius 3.5
  dimension "d256" = -0.5
  dimension "d257" = -0.5
  dimension "d258" = -0.5
  dimension "d259" = -0.5
  dimension "d260" = 0.5
extrude "Extrude35" add sketch "Sketch29" along normal blind 0.35 contours L22 L23 L24 | L25 L26 L27 | L28 L29 L30 | L31 L32 L33 | A7
sketch "Sketch30" plane through (-2.5, 0, 0) normal (-1, 0, 0) x (0, 0, 1)
  line L0 (35.5, 59.8175) -> (35.5, 45.1825)
  line L1 (35.5, 45.1825) -> (26.719, 52.5)
  line L2 (26.719, 52.5) -> (35.5, 59.8175)
  line L3 (9.5, 59.8175) -> (18.281, 52.5)
  line L4 (18.281, 52.5) -> (9.5, 45.1825)
  line L5 (9.5, 45.1825) -> (9.5, 59.8175)
  line L6 (29.8175, 39.5) -> (15.1825, 39.5)
  line L7 (15.1825, 39.5) -> (22.5, 48.281)
  line L8 (22.5, 48.281) -> (29.8175, 39.5)
  line L9 (22.5, 56.719) -> (15.1825, 65.5)
  line L10 (15.1825, 65.5) -> (29.8175, 65.5)
  line L11 (29.8175, 65.5) -> (22.5, 56.719)
  circle A0 centre (38.5, 65) radius 0.9
  circle A1 centre (6.5, 65) radius 0.9
  circle A2 centre (22.5, 52.5) radius 3
  arc A3 (23.5, 4) -> (26, 1.5) centre (26, 4) ccw
  line L12 (23.5, 4) -> (23.5, 8.5)
  line L13 (23.5, 8.5) -> (6, 8.5)
  arc A4 (3.5, 11) -> (6, 8.5) centre (6, 11) ccw
  line L14 (3.5, 11) -> (3.5, 19)
  arc A5 (6, 21.5) -> (3.5, 19) centre (6, 19) ccw
  line L15 (6, 21.5) -> (26.5, 21.5)
  line L16 (26.5, 21.5) -> (26.5, 24)
  arc A6 (29, 26.5) -> (26.5, 24) centre (29, 24) ccw
  line L17 (29, 26.5) -> (39, 26.5)
  arc A7 (41.5, 24) -> (39, 26.5) centre (39, 24) ccw
  line L18 (41.5, 24) -> (41.5, 11)
  arc A8 (39, 8.5) -> (41.5, 11) centre (39, 11) ccw
  line L19 (39, 8.5) -> (36.5, 8.5)
  line L20 (36.5, 8.5) -> (36.5, 4)
  arc A9 (34, 1.5) -> (36.5, 4) centre (34, 4) ccw
  line L21 (34, 1.5) -> (46, 1.5)
  line L22 (46, 1.5) -> (46, 68.5)
  line L23 (46, 68.5) -> (-1.4, 68.5)
  line L24 (-1.4, 68.5) -> (-1.4, 1.5)
  line L25 (-1.4, 1.5) -> (26, 1.5)
  circle A10 centre (22.5, 52.5) radius 3.5
  dimension "d263" = 0.5
extrude "Extrude36" add sketch "Sketch30" along normal blind 0.35 contours A10
sketch "Sketch31" plane through (0, 0, -2.5) normal (0, 0, -1) x (-1, 0, 0)
  line L0 (-18.281, 17.5) -> (-9.5, 24.8175)
  line L1 (-9.5, 24.8175) -> (-9.5, 10.1825)
  line L2 (-9.5, 10.1825) -> (-18.281, 17.5)
  line L3 (-15.1825, 39.5) -> (-29.8175, 39.5)
  line L4 (-29.8175, 39.5) -> (-22.5, 48.281)
  line L5 (-22.5, 48.281) -> (-15.1825, 39.5)
  line L6 (-29.8175, 65.5) -> (-15.1825, 65.5)
  line L7 (-15.1825, 65.5) -> (-22.5, 56.719)
  line L8 (-22.5, 56.719) -> (-29.8175, 65.5)
  line L9 (-22.5, 21.719) -> (-29.8175, 30.5)
  line L10 (-29.8175, 30.5) -> (-15.1825, 30.5)
  line L11 (-15.1825, 30.5) -> (-22.5, 21.719)
  line L12 (-15.1825, 4.5) -> (-29.8175, 4.5)
  line L13 (-29.8175, 4.5) -> (-22.5, 13.281)
  line L14 (-22.5, 13.281) -> (-15.1825, 4.5)
  line L15 (-18.281, 52.5) -> (-9.5, 59.8175)
  line L16 (-9.5, 59.8175) -> (-9.5, 45.1825)
  line L17 (-9.5, 45.1825) -> (-18.281, 52.5)
  line L18 (-35.5, 59.8175) -> (-26.719, 52.5)
  line L19 (-26.719, 52.5) -> (-35.5, 45.1825)
  line L20 (-35.5, 45.1825) -> (-35.5, 59.8175)
  line L21 (-35.5, 10.1825) -> (-35.5, 24.8175)
  line L22 (-35.5, 24.8175) -> (-26.719, 17.5)
  line L23 (-26.719, 17.5) -> (-35.5, 10.1825)
  circle A0 centre (-22.5, 52.5) radius 3
  circle A1 centre (-22.5, 17.5) radius 3
  line L24 (-37.85, 1.5) -> (-37.85, 2)
  line L25 (-37.85, 2) -> (-33.85, 2)
  line L26 (-33.85, 2) -> (-33.85, 1.5)
  line L27 (-33.85, 1.5) -> (1, 1.5)
  line L28 (1, 1.5) -> (1, 68.5)
  line L29 (1, 68.5) -> (-46.35, 68.5)
  line L30 (-46.35, 68.5) -> (-46.35, 1.5)
  line L31 (-46.35, 1.5) -> (-37.85, 1.5)
  circle A2 centre (-22.5, 52.5) radius 3.5
  dimension "d266" = 0.5
extrude "Extrude37" add sketch "Sketch31" along normal blind 0.35 contours A2
sketch "Sketch32" plane through (0, 0, -2.5) normal (0, 0, -1) x (-1, 0, 0)
  circle A0 centre (-22.5, 52.5) radius 3.5
  line L0 (-18.281, 17.5) -> (-9.5, 24.8175)
  line L1 (-9.5, 24.8175) -> (-9.5, 10.1825)
  line L2 (-9.5, 10.1825) -> (-18.281, 17.5)
  line L3 (-15.1825, 39.5) -> (-29.8175, 39.5)
  line L4 (-29.8175, 39.5) -> (-22.5, 48.281)
  line L5 (-22.5, 48.281) -> (-15.1825, 39.5)
  line L6 (-29.8175, 65.5) -> (-15.1825, 65.5)
  line L7 (-15.1825, 65.5) -> (-22.5, 56.719)
  line L8 (-22.5, 56.719) -> (-29.8175, 65.5)
  line L9 (-22.5, 21.719) -> (-29.8175, 30.5)
  line L10 (-29.8175, 30.5) -> (-15.1825, 30.5)
  line L11 (-15.1825, 30.5) -> (-22.5, 21.719)
  line L12 (-15.1825, 4.5) -> (-29.8175, 4.5)
  line L13 (-29.8175, 4.5) -> (-22.5, 13.281)
  line L14 (-22.5, 13.281) -> (-15.1825, 4.5)
  line L15 (-18.281, 52.5) -> (-9.5, 59.8175)
  line L16 (-9.5, 59.8175) -> (-9.5, 45.1825)
  line L17 (-9.5, 45.1825) -> (-18.281, 52.5)
  line L18 (-35.5, 59.8175) -> (-26.719, 52.5)
  line L19 (-26.719, 52.5) -> (-35.5, 45.1825)
  line L20 (-35.5, 45.1825) -> (-35.5, 59.8175)
  line L21 (-35.5, 10.1825) -> (-35.5, 24.8175)
  line L22 (-35.5, 24.8175) -> (-26.719, 17.5)
  line L23 (-26.719, 17.5) -> (-35.5, 10.1825)
  circle A1 centre (-22.5, 17.5) radius 3
  line L24 (-37.85, 1.5) -> (-37.85, 2)
  line L25 (-37.85, 2) -> (-33.85, 2)
  line L26 (-33.85, 2) -> (-33.85, 1.5)
  line L27 (-33.85, 1.5) -> (1, 1.5)
  line L28 (1, 1.5) -> (1, 68.5)
  line L29 (1, 68.5) -> (-46.35, 68.5)
  line L30 (-46.35, 68.5) -> (-46.35, 1.5)
  line L31 (-46.35, 1.5) -> (-37.85, 1.5)
  circle A2 centre (-22.5, 17.5) radius 3.5
  dimension "d269" = 0.5
extrude "Extrude38" add sketch "Sketch32" along normal blind 0.35 contours A2